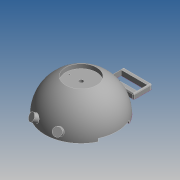
# Autodesk Inventor part: body_face
Saved by Autodesk Inventor 2017 (Build 210142000, 142)
## iProperties
Created: 2018-10-05
Part Number: body_face
Material: Générique
Document SubType Name: Modeling
Designer: Gilles Mottiez
Density: 1 g/cm^3
Appearance: Par défaut
Author: Gilles Mottiez
Autodesk Inventor part; units mm, degrees
ref_plane "YZ Plane" through (0, 0, 0) normal (1, 0, 0) x (0, 1, 0)
ref_plane "XZ Plane" through (0, 0, 0) normal (0, 1, 0) x (-1, 0, 0)
ref_plane "XY Plane" through (0, 0, 0) normal (0, 0, 1) x (1, 0, 0)
sketch "Sketch1" plane through (0, 0, 0) normal (0, 0, 1) x (1, 0, 0)
  circle A0 centre (0, 0) radius 70 construction
  line L0 (-70, 0) -> (70, 0) construction
  arc A1 (70, 0) -> (-70, 0) centre (0, 0) ccw
  line L1 (-70, 0) -> (70, 0)
  dimension "d0" = 140
  constraints: 4 end point, 4 point on circle, 2 centre point, 2 coincident, 1 collinear, 1 concentric, 1 horizontal, 1 midpoint
  measures "d0" diameter of A0
revolve "Révolution1" add sketch "Sketch1" angle 180 about axis through (-70, 0, 0) along (1, 0, 0)
sketch "Esquisse2" plane through (0, 0, 0) normal (1, 0, 0) x (0, 1, 0)
  line L0 (-70, 0) -> (70, 0) construction
  circle A0 centre (0, 0) radius 67 construction
  arc A1 (67, 0) -> (-67, 0) centre (0, 0) ccw
  line L1 (67, 0) -> (-67, 0)
  dimension "d2" = 134
  constraints: 4 point on circle, 2 centre point, 2 concentric, 2 end point, 2 point on line, 1 coincident, 1 collinear
  measures "d2" diameter of A0
revolve "Révolution2" cut sketch "Esquisse2" angle 360 about axis through (0, 67, 0) along (0, -1, 0)
sketch "Esquisse3" plane through (0, 0, 0) normal (1, 0, 0) x (0, 1, 0)
  line L0 (67, 0) -> (-67, 0) construction
  line L1 (-70, 0) -> (70, 0) construction
  arc A0 (70, 0) -> (-70, 0) centre (0, 0) ccw construction
  line L2 (30, 0) -> (-30, 0)
  line L3 (-30, 0) -> (-30, 5.5)
  line L4 (-30, 5.5) -> (30, 5.5)
  line L5 (30, 5.5) -> (30, 0)
  point P0 (0, 0)
  point P1 (0, 0)
  point P2 (0, 5.5)
  dimension "d4" = 60
  dimension "d5" = 5.5
  constraints: 8 end point, 2 midpoint, 2 parallel, 1 horizontal, 1 perpendicular, 1 point on line, 1 vertical alignment
  measures "d4" distance of L3.end L4.end
  measures "d5" distance of L4.end L2.start
extrude "Extrusion1" cut sketch "Esquisse3" along normal through all both and the other way through all
sketch "Esquisse4" plane through (0, 0, 0) normal (0, 0, -1) x (-1, 0, 0)
  line L0 (-63.2456, 30) -> (-59.9083, 30) construction
  arc A0 (59.9083, 30) -> (-59.9083, 30) centre (0, 0) ccw construction
  line L1 (59.9083, 30) -> (63.2456, 30) construction
  arc A1 (63.2456, 30) -> (-63.2456, 30) centre (0, 0) ccw construction
  arc A2 (-59.9083, -30) -> (59.9083, -30) centre (0, 0) ccw construction
  line L2 (-59.9083, -30) -> (-63.2456, -30) construction
  arc A3 (-63.2456, -30) -> (63.2456, -30) centre (0, 0) ccw construction
  line L3 (63.2456, -30) -> (59.9083, -30) construction
  arc A4 (-59.9083, -30) -> (59.9083, -30) centre (0, 0) ccw construction
  arc A5 (-59.6553, 30) -> (-59.6553, -30) centre (0, 0) ccw construction
  line L4 (-63.006, 30) -> (-59.6553, 30) construction
  arc A6 (-63.006, 30) -> (-63.006, -30) centre (0, 0) ccw construction
  line L5 (-63.006, -30) -> (-59.6553, -30) construction
  arc A7 (59.6553, -30) -> (59.6553, 30) centre (0, 0) ccw construction
  line L6 (59.6553, -30) -> (63.006, -30) construction
  arc A8 (63.006, -30) -> (63.006, 30) centre (0, 0) ccw construction
  line L7 (59.6553, 30) -> (63.006, 30) construction
  line L8 (0, 0) -> (-49.4975, 49.4975) construction
  line L9 (0, 0) -> (-69.7836, 0) construction
  circle A9 centre (0, 0) radius 63 construction
  circle A10 centre (-44.5477, 44.5477) radius 4 construction
  line L10 (-41.6309, 47.2849) -> (-44.5602, 50.0339)
  line L11 (-47.2849, 41.6309) -> (-50.2031, 44.3694)
  arc A11 (-44.5602, 50.0339) -> (-50.2031, 44.3694) centre (0, 0) ccw
  arc A12 (-47.2849, 41.6309) -> (-41.6309, 47.2849) centre (-44.5477, 44.5477) ccw
  dimension "d8" = 45
  dimension "d9" = 126
  dimension "d10" = 8
  constraints: 13 point on circle, 8 end point, 4 centre point, 2 concentric, 2 tangent, 1 coincident, 1 parallel, 1 point on line
  measures "d8" angle of L8 L9
  measures "d9" diameter of A9
  measures "d10" diameter of A10
extrude "Extrusion2" add sketch "Esquisse4" against normal up to surface
pattern_circular "Réseau circulaire1" count 4 over 360 about axis through (0, 0, 0) along (0, 0, 1) of "Extrusion2"
sketch "Esquisse6" plane through (0, 0, 0) normal (0, 0, -1) x (-1, 0, 0)
  line L0 (-63.2456, 30) -> (-59.9083, 30) construction
  arc A0 (-50.2031, 44.3694) -> (-59.9083, 30) centre (0, 0) ccw construction
  line L1 (-50.2031, 44.3694) -> (-47.2849, 41.6309) construction
  arc A1 (-47.2849, 41.6309) -> (-41.6309, 47.2849) centre (-44.5477, 44.5477) ccw construction
  line L2 (-41.6309, 47.2849) -> (-44.5602, 50.0339) construction
  arc A2 (44.3694, 50.2031) -> (-44.5602, 50.0339) centre (0, 0) ccw construction
  line L3 (44.3694, 50.2031) -> (41.6309, 47.2849) construction
  arc A3 (41.6309, 47.2849) -> (47.2849, 41.6309) centre (44.5477, 44.5477) ccw construction
  line L4 (47.2849, 41.6309) -> (50.0339, 44.5602) construction
  arc A4 (59.9083, 30) -> (50.0339, 44.5602) centre (0, 0) ccw construction
  line L5 (59.9083, 30) -> (63.2456, 30) construction
  arc A5 (63.2456, 30) -> (-63.2456, 30) centre (0, 0) ccw construction
  circle A6 centre (-44.5477, 44.5477) radius 2.5
  dimension "d19" = 5
  constraints: 1 centre point, 1 coincident
  measures "d19" diameter of A6
extrude "Extrusion4" cut sketch "Esquisse6" against normal blind 4
pattern_circular "Réseau circulaire2" count 4 over 360 about axis through (0, 0, 0) along (0, 0, 1) of "Extrusion4"
sketch "Esquisse7" plane through (0, 0, 0) normal (0, 0, 1) x (1, 0, 0)
  arc A0 (-63.2456, -30) -> (63.2456, -30) centre (0, 0) ccw construction
  line L0 (50.0339, -44.5602) -> (47.2849, -41.6309) construction
  line L1 (41.6309, -47.2849) -> (44.3694, -50.2031) construction
  arc A1 (-44.5602, -50.0339) -> (44.3694, -50.2031) centre (0, 0) ccw construction
  line L2 (-44.5602, -50.0339) -> (-41.6309, -47.2849) construction
  line L3 (-47.2849, -41.6309) -> (-50.2031, -44.3694) construction
  arc A2 (-59.9083, -30) -> (-50.2031, -44.3694) centre (0, 0) ccw construction
  line L4 (-59.9083, -30) -> (-59.6553, -30) construction
  arc A3 (-59.6553, 30) -> (-59.6553, -30) centre (0, 0) ccw construction
  line L5 (-59.6553, 30) -> (-59.9083, 30) construction
  arc A4 (-50.0339, 44.5602) -> (-59.9083, 30) centre (0, 0) ccw construction
  line L6 (-50.0339, 44.5602) -> (-47.2849, 41.6309) construction
  line L7 (-41.6309, 47.2849) -> (-44.3694, 50.2031) construction
  arc A5 (44.5602, 50.0339) -> (-44.3694, 50.2031) centre (0, 0) ccw construction
  line L8 (44.5602, 50.0339) -> (41.6309, 47.2849) construction
  line L9 (47.2849, 41.6309) -> (50.2031, 44.3694) construction
  arc A6 (59.9083, 30) -> (50.2031, 44.3694) centre (0, 0) ccw construction
  line L10 (59.9083, 30) -> (59.6553, 30) construction
  arc A7 (59.6553, -30) -> (59.6553, 30) centre (0, 0) ccw construction
  line L11 (59.6553, -30) -> (59.9083, -30) construction
  arc A8 (50.0339, -44.5602) -> (59.9083, -30) centre (0, 0) ccw construction
  line L12 (50, -70) -> (-50, -70) construction
  point P0 (0, -70)
  point P1 (0, -70)
  dimension "d25" = 100
  constraints: 2 end point, 1 coincident, 1 horizontal, 1 midpoint, 1 point on circle, 1 vertical alignment, 4 other
  measures "d25" distance of L12.start L12.end
ref_plane "Plan de construction1" through (50, -70, 0) normal (0, -0.8660254, 0.5) x (-1, 0, 0)
ref_plane "Plan de construction2" through (50, -78.6603, 5) normal (0, -0.8660254, 0.5) x (-1, 0, 0)
sketch "Esquisse9" plane through (50, -78.6603, 5) normal (0, -0.8660254, 0.5) x (-1, 0, 0)
  line L0 (0, 0) -> (100, 0) construction
  ellipse E0 centre (50, -50) end of major axis (113.2456, -50) minor radius 54.7723 (-13.2456, -50) -> (-13.006, -54.7631) ccw construction
  ellipse E1 centre (50, -35) end of major axis (120, -35) minor radius 35 (-13.2456, -50) -> (113.2456, -50) ccw construction
  ellipse E2 centre (50, -50) end of major axis (113.2456, -50) minor radius 54.7723 (113.006, -54.7631) -> (113.2456, -50) ccw construction
  ellipse E3 centre (50, -39.7631) end of major axis (119.7836, -39.7631) minor radius 34.8918 (113.006, -54.7631) -> (113.006, -24.7631) ccw construction
  ellipse E4 centre (50, -20) end of major axis (113.2456, -20) minor radius 54.7723 (113.006, -24.7631) -> (113.2456, -20) ccw construction
  ellipse E5 centre (50, -35) end of major axis (120, -35) minor radius 35 (113.2456, -20) -> (-13.2456, -20) ccw construction
  ellipse E6 centre (50, -20) end of major axis (113.2456, -20) minor radius 54.7723 (-13.2456, -20) -> (-13.006, -24.7631) ccw construction
  ellipse E7 centre (50, -39.7631) end of major axis (119.7836, -39.7631) minor radius 34.8918 (-13.006, -24.7631) -> (-13.006, -54.7631) ccw construction
  line L1 (75, 0) -> (75, -50) construction
  line L2 (25, 0) -> (25, -50) construction
  point P0 (50, -35)
  point P1 (50, 0)
  dimension "d32" = 50
  dimension "d34" = 25
  dimension "d40" = 50
  dimension "d41" = 25
  constraints: 4 end point, 2 point on line, 2 vertical, 8 other
  measures "d32" distance of L1.start L1.end
  measures "d34" distance from line of point (50, 0) L1
  measures "d40" distance of L2.start L2.end
  measures "d41" distance from line of L2 point (50, -20)
ref_plane "Plan de construction3" through (-25, -78.6603, 5) normal (-0.3420201, -0.8137977, 0.4698463) x (0, 0.5, 0.8660254)
sketch "Esquisse10" plane through (-25, -78.6603, 5) normal (-0.3420201, -0.8137977, 0.4698463) x (0, 0.5, 0.8660254)
  ellipse E0 centre (50, 9.5477) end of major axis (17.7652, 63.962) minor radius 51.4691 (50, -49.8837) -> (54.7631, -50.5991) ccw construction
  ellipse E1 centre (35, 0.6618) end of major axis (48.5607, 69.3357) minor radius 32.8892 (50, -49.8837) -> (50, 68.9791) ccw construction
  ellipse E2 centre (50, 9.5477) end of major axis (17.7652, 63.962) minor radius 51.4691 (54.7631, 67.8134) -> (50, 68.9791) ccw construction
  ellipse E3 centre (39.7631, -0.2788) end of major axis (53.2819, 68.1828) minor radius 32.7876 (54.7631, 67.8134) -> (24.7631, 50.0415) ccw construction
  ellipse E4 centre (20, -8.2242) end of major axis (-12.2348, 46.1901) minor radius 51.4691 (24.7631, 50.0415) -> (20, 51.2072) ccw construction
  ellipse E5 centre (35, 0.6618) end of major axis (48.5607, 69.3357) minor radius 32.8892 (20, 51.2072) -> (20, -67.6556) ccw construction
  ellipse E6 centre (20, -8.2242) end of major axis (-12.2348, 46.1901) minor radius 51.4691 (20, -67.6556) -> (24.7631, -68.371) ccw construction
  ellipse E7 centre (39.7631, -0.2788) end of major axis (53.2819, 68.1828) minor radius 32.7876 (24.7631, -68.371) -> (54.7631, -50.5991) ccw construction
  line L0 (0, 0) -> (50, 0) construction
  line L1 (0, -70.4769) -> (0, 23.4923) construction
  circle A0 centre (15, 0) radius 7.5
  point P0 (35, 0.6618)
  dimension "d36" = 15
  dimension "d37" = 15
  constraints: 1 centre point, 1 point on line, 8 other
  measures "d36" diameter of A0
  measures "d37" distance from line of L1 A0.centre
extrude "Extrusion5" add sketch "Esquisse10" against normal up to surface
ref_plane "Plan de construction4" through (25, -78.6603, 5) normal (0.3420201, -0.8137977, 0.4698463) x (0, 0.5, 0.8660254)
sketch "Esquisse11" plane through (25, -78.6603, 5) normal (0.3420201, -0.8137977, 0.4698463) x (0, 0.5, 0.8660254)
  line L0 (0, 0) -> (50, 0) construction
  line L1 (0, -23.4923) -> (0, 70.4769) construction
  circle A0 centre (15, 0) radius 7.5
  point P0 (35, -0.6618)
  dimension "d43" = 15
  dimension "d44" = 15
  constraints: 1 centre point, 1 point on line
  measures "d43" diameter of A0
  measures "d44" distance from line of L1 A0.centre
extrude "Extrusion6" add sketch "Esquisse11" against normal up to surface
sketch "Esquisse12" plane through (0, 0, 0) normal (1, 0, 0) x (0, 1, 0)
  arc A0 (67, 0) -> (-67, 0) centre (0, 0) ccw construction
  arc A1 (70, 0) -> (-70, 0) centre (0, 0) ccw construction
  line L0 (0, -14.3596) -> (0, 86.1577) construction
  ellipse E0 centre (4.1003, 0) end of major axis (4.1003, -66.7315) minor radius 48.6605 (-41.6309, 22.8035) -> (-44.5602, 0) ccw construction
  ellipse E1 centre (-1.3686, 0) end of major axis (-1.3686, 66.9701) minor radius 48.8345 (-47.2849, 22.8035) -> (-50.2031, 0) ccw construction
  line L1 (-50.0339, 0) -> (-50.2031, 0) construction
  ellipse E2 centre (-4.3693, 0) end of major axis (-4.3693, 66.7315) minor radius 45.6646 (-47.2849, 22.8035) -> (-50.0339, 0) ccw construction
  ellipse E3 centre (1.4584, 0) end of major axis (1.4584, -66.9701) minor radius 45.8278 (-41.6309, 22.8035) -> (-44.3694, 0) ccw construction
  line L2 (-30, 0) -> (-44.3694, 0) construction
  line L3 (-30, 0) -> (-30, 5.5) construction
  line L4 (-30, 5.5) -> (30, 5.5) construction
  line L5 (30, 5.5) -> (30, 0) construction
  line L6 (44.5602, 0) -> (30, 0) construction
  ellipse E4 centre (-4.1003, 0) end of major axis (-4.1003, 66.7315) minor radius 48.6605 (44.5602, 0) -> (41.6309, 22.8035) ccw construction
  ellipse E5 centre (1.3686, 0) end of major axis (1.3686, -66.9701) minor radius 48.8345 (50.2031, 0) -> (47.2849, 22.8035) ccw construction
  line L7 (50.0339, 0) -> (50.2031, 0) construction
  ellipse E6 centre (4.3693, 0) end of major axis (4.3693, -66.7315) minor radius 45.6646 (50.0339, 0) -> (47.2849, 22.8035) ccw construction
  ellipse E7 centre (-1.4584, 0) end of major axis (-1.4584, 66.9701) minor radius 45.8278 (44.3694, 0) -> (41.6309, 22.8035) ccw construction
  line L8 (30, 0) -> (44.3694, 0) construction
  line L9 (30, 0) -> (30, 5.5) construction
  line L10 (30, 5.5) -> (-30, 5.5) construction
  line L11 (-30, 5.5) -> (-30, 0) construction
  line L12 (-44.5602, 0) -> (-30, 0) construction
  line L13 (0, 47) -> (47.7493, 47)
  arc A2 (47.7493, 47) -> (0, 67) centre (0, 0) ccw
  line L14 (0, 67) -> (0, 47)
  point P0 (0, 0)
  point P1 (4, 66.8805)
  point P2 (-4, 66.8805)
  dimension "d48" = 20
  constraints: 4 end point, 4 horizontal alignment, 4 point on circle, 2 point on line, 1 centre point, 1 collinear, 1 concentric, 1 horizontal, 8 other
  measures "d48" distance from line of L14.start L13
revolve "Révolution3" add sketch "Esquisse12" angle 360 about axis through (0, 0, 67) along (0, 0, -1)
sketch "Esquisse13" plane through (0, 0, 0) normal (1, 0, 0) x (0, 1, 0)
  line L0 (30, 5.5) -> (30, 0) construction
  line L1 (30, 0) -> (30, 0) construction
  line L2 (30, 0) -> (30, 5.5) construction
  line L3 (30, 5.5) -> (-30, 5.5) construction
  line L4 (-30, 5.5) -> (-30, 0) construction
  line L5 (-30, 0) -> (-30, 0) construction
  line L6 (-30, 0) -> (-30, 5.5) construction
  line L7 (-30, 5.5) -> (30, 5.5) construction
  line L8 (47.7493, 47) -> (-47.7493, 47) construction
  line L9 (0, -15) -> (0, 90) construction
  arc A0 (70, 0) -> (-70, 0) centre (0, 0) ccw construction
  line L10 (0, 55) -> (30, 55) construction
  line L11 (30, 55) -> (30, 75) construction
  line L12 (30, 75) -> (0, 75) construction
  line L13 (0, 75) -> (0, 55) construction
  line L14 (0, 55) -> (30, 55)
  line L15 (30, 55) -> (30, 63.2456)
  arc A1 (30, 63.2456) -> (0, 70) centre (0, 0) ccw
  line L16 (0, 55) -> (0, 70)
  point P0 (0, 0)
  dimension "d50" = 8
  dimension "d51" = 30
  dimension "d52" = 20
  constraints: 14 end point, 4 point on circle, 3 point on line, 2 collinear, 2 parallel, 1 centre point, 1 concentric, 1 horizontal, 1 perpendicular, 2 other
  measures "d50" distance between parallel lines of L10 L8
  measures "d51" distance between parallel lines of L13 L11
  measures "d52" distance of L10.end L11.end
revolve "Révolution4" cut sketch "Esquisse13" angle 360 about axis through (0, 0, 55) along (0, 0, 1)
sketch "Esquisse15" plane through (0, 0, 55) normal (0, 0, 1) x (1, 0, 0)
  point P0 (0, 0)
  point P1 (-23, 0)
  dimension "d57" = 23
  constraints: 1 horizontal alignment
  measures "d57" distance of point (-23, 0) point (0, 0)
hole "Perçage1" at (-23, 0, 55) direction (0, 0, -1) diameter 3 depth 8 tip angle 118
sketch "Esquisse16" plane through (0, 0, 0) normal (1, 0, 0) x (0, 1, 0)
  line L0 (-30, 63.2456) -> (30, 63.2456) construction
  line L1 (30, 5.5) -> (30, 0) construction
  line L2 (30, 0) -> (30, 0) construction
  line L3 (30, 0) -> (30, 5.5) construction
  line L4 (30, 5.5) -> (-30, 5.5) construction
  line L5 (-30, 5.5) -> (-30, 0) construction
  line L6 (-30, 0) -> (-30, 0) construction
  line L7 (-30, 0) -> (-30, 5.5) construction
  line L8 (-30, 5.5) -> (30, 5.5) construction
  line L9 (47.7493, 47) -> (-47.7493, 47) construction
  line L10 (4, 47) -> (-4, 47) construction
  line L11 (-4, 55) -> (4, 55) construction
  line L12 (0, -13.1244) -> (0, 78.7461) construction
  line L13 (0, 41) -> (6, 41) construction
  line L14 (6, 41) -> (6, 47) construction
  line L15 (6, 47) -> (0, 47) construction
  line L16 (0, 47) -> (0, 41) construction
  arc A0 (11, 47) -> (6, 42) centre (11, 42) ccw construction
  line L17 (0, 47) -> (11, 47)
  line L18 (6, 41) -> (0, 41)
  line L19 (6, 41) -> (6, 42)
  arc A1 (11, 47) -> (6, 42) centre (11, 42) ccw
  line L20 (0, 41) -> (0, 47)
  point P0 (0, 0)
  dimension "d65" = 12
  dimension "d67" = 5
  dimension "d68" = 6
  constraints: 16 end point, 4 collinear, 4 point on circle, 4 point on line, 3 tangent, 2 centre point, 2 parallel, 1 concentric, 1 horizontal, 1 perpendicular, 2 other
  measures "d65" diameter of L14 L20
  measures "d67" radius of A0
  measures "d68" distance between parallel lines of L17 L13
revolve "Révolution5" add sketch "Esquisse16" angle 360 about axis through (0, 0, 41) along (0, 0, 1)
sketch "Esquisse17" plane through (0, 0, 41) normal (0, 0, -1) x (-1, 0, 0)
  circle A0 centre (0, 0) radius 4
  point P0 (0, 0)
  dimension "d70" = 8
  constraints: 1 centre point, 1 coincident
  measures "d70" diameter of A0
extrude "Extrusion8" cut sketch "Esquisse17" against normal through all
sketch "Esquisse19" plane through (0, 0, 0) normal (0, 0, -1) x (-1, 0, 0)
  circle A0 centre (44.5477, 44.5477) radius 2.5 construction
  circle A1 centre (-44.5477, 44.5477) radius 2.5 construction
  line L0 (-63.2456, 30) -> (-59.9083, 30) construction
  arc A2 (-50.2031, 44.3694) -> (-59.9083, 30) centre (0, 0) ccw construction
  line L1 (-50.2031, 44.3694) -> (-47.2849, 41.6309) construction
  arc A3 (-47.2849, 41.6309) -> (-41.6309, 47.2849) centre (-44.5477, 44.5477) ccw construction
  line L2 (-41.6309, 47.2849) -> (-44.5602, 50.0339) construction
  arc A4 (44.3694, 50.2031) -> (-44.5602, 50.0339) centre (0, 0) ccw construction
  line L3 (44.3694, 50.2031) -> (41.6309, 47.2849) construction
  arc A5 (41.6309, 47.2849) -> (47.2849, 41.6309) centre (44.5477, 44.5477) ccw construction
  line L4 (47.2849, 41.6309) -> (50.0339, 44.5602) construction
  arc A6 (59.9083, 30) -> (50.0339, 44.5602) centre (0, 0) ccw construction
  line L5 (59.9083, 30) -> (63.2456, 30) construction
  arc A7 (63.2456, 30) -> (-63.2456, 30) centre (0, 0) ccw construction
  line L6 (0, 0) -> (0, 70) construction
  line L7 (-27.5, 110) -> (27.5, 110) construction
  line L8 (27.5, 110) -> (27.5, 75) construction
  line L9 (27.5, 75) -> (-27.5, 75) construction
  line L10 (-27.5, 75) -> (-27.5, 110) construction
  line L11 (-10, 75) -> (10, 75) construction
  line L12 (10, 75) -> (10, 69.282) construction
  line L13 (10, 69.282) -> (-10, 69.282) construction
  line L14 (-10, 69.282) -> (-10, 75) construction
  line L15 (-10, 69.282) -> (-10, 75)
  line L16 (-10, 75) -> (-27.5, 75)
  line L17 (-27.5, 75) -> (-27.5, 110)
  line L18 (-27.5, 110) -> (27.5, 110)
  line L19 (27.5, 110) -> (27.5, 75)
  line L20 (27.5, 75) -> (10, 75)
  line L21 (10, 75) -> (10, 69.282)
  line L22 (10, 69.282) -> (-10, 69.282)
  dimension "d79" = 55
  dimension "d80" = 35
  dimension "d81" = 75
  dimension "d82" = 20
  constraints: 34 end point, 7 collinear, 4 parallel, 3 horizontal, 2 perpendicular, 2 point on circle, 1 point on line, 2 other
  measures "d79" distance of L8.end L9.end
  measures "d80" distance of L7.end L8.end
  measures "d81" distance from line of point (0, 0) L9
  measures "d82" distance of L12.end L13.end
extrude "Extrusion10" add sketch "Esquisse19" against normal blind 10
thicken "Epaississement2" operation add thickness 1 both sides no extend neighbours yes toward (0, -1, 0) faces at (8.0177, 69.282, 8.0177)
thicken "Epaississement3" operation add thickness 1 both sides no extend neighbours yes toward (0, -1, 0) faces at (-8.0177, 69.282, 8.0177)
fillet "Congé1" radius 2 14 edges at (10, 71.7783, 10) (10, 69.1004, 5.0131) (-10, 71.7783, 10) (0, 69.282, 10) (-10, 69.1004, 5.0131) (-18.75, 75, 10) (-27.5, 92.5, 10) (0, 110, 10) (27.5, 92.5, 10) (18.75, 75, 10) (27.5, 110, 5) (-27.5, 110, 5) (27.5, 75, 5) (-27.5, 75, 5)
sketch "Esquisse20" plane through (25.5, 110, 0) normal (0, 0, -1) x (-1, 0, 0)
  arc A0 (0, 0) -> (-2, -2) centre (0, -2) ccw construction
  line L0 (-2, -2) -> (-2, -33) construction
  arc A1 (-2, -33) -> (0, -35) centre (0, -33) ccw construction
  line L1 (0, -35) -> (15.5, -35) construction
  line L2 (15.5, -35) -> (15.5, -39.007) construction
  arc A2 (13.8333, -40.9791) -> (15.5, -39.007) centre (13.5, -39.007) ccw construction
  arc A3 (13.8333, -40.9791) -> (-37.7456, -80) centre (25.5, -110) ccw construction
  line L3 (-37.7456, -80) -> (-34.4083, -80) construction
  arc A4 (-24.7031, -65.6306) -> (-34.4083, -80) centre (25.5, -110) ccw construction
  line L4 (-24.7031, -65.6306) -> (-21.7849, -68.3691) construction
  arc A5 (-21.7849, -68.3691) -> (-16.1309, -62.7151) centre (-19.0477, -65.4523) ccw construction
  line L5 (-16.1309, -62.7151) -> (-19.0602, -59.9661) construction
  arc A6 (69.8694, -59.7969) -> (-19.0602, -59.9661) centre (25.5, -110) ccw construction
  line L6 (69.8694, -59.7969) -> (67.1309, -62.7151) construction
  arc A7 (67.1309, -62.7151) -> (72.7849, -68.3691) centre (70.0477, -65.4523) ccw construction
  line L7 (72.7849, -68.3691) -> (75.5339, -65.4398) construction
  arc A8 (85.4083, -80) -> (75.5339, -65.4398) centre (25.5, -110) ccw construction
  line L8 (85.4083, -80) -> (88.7456, -80) construction
  arc A9 (88.7456, -80) -> (37.1667, -40.9791) centre (25.5, -110) ccw construction
  arc A10 (35.5, -39.007) -> (37.1667, -40.9791) centre (37.5, -39.007) ccw construction
  line L9 (35.5, -39.007) -> (35.5, -35) construction
  line L10 (35.5, -35) -> (51, -35) construction
  arc A11 (51, -35) -> (53, -33) centre (51, -33) ccw construction
  line L11 (53, -33) -> (53, -2) construction
  arc A12 (53, -2) -> (51, 0) centre (51, -2) ccw construction
  line L12 (51, 0) -> (0, 0) construction
  circle A13 centre (-19.0477, -65.4523) radius 2.5 construction
  circle A14 centre (70.0477, -65.4523) radius 2.5 construction
  line L13 (0, -7) -> (51, -7)
  line L14 (51, -7) -> (51, -27)
  line L15 (51, -27) -> (0, -27)
  line L16 (0, -27) -> (0, -7)
  line L17 (25.5, 0) -> (25.5, -43) construction
  dimension "d90" = 51
  dimension "d91" = 20
  dimension "d92" = 7
  constraints: 10 end point, 2 parallel, 1 horizontal, 1 midpoint, 1 perpendicular, 1 point on circle, 1 vertical, 1 other
  measures "d90" distance of L14.end L15.end
  measures "d91" distance of L13.end L14.end
  measures "d92" distance between parallel lines of L12 L13
extrude "Extrusion11" cut sketch "Esquisse20" against normal through all
sketch "Esquisse21" plane through (25.5, 110, 0) normal (0, 0, -1) x (-1, 0, 0)
  line L0 (0, -27) -> (0, -7) construction
  line L1 (0, -7) -> (51, -7) construction
  line L2 (51, -7) -> (51, -27) construction
  line L3 (51, -27) -> (0, -27) construction
  arc A0 (0, 0) -> (-2, -2) centre (0, -2) ccw construction
  line L4 (-2, -2) -> (-2, -33) construction
  arc A1 (-2, -33) -> (0, -35) centre (0, -33) ccw construction
  line L5 (0, -35) -> (15.5, -35) construction
  line L6 (15.5, -35) -> (15.5, -39.007) construction
  arc A2 (13.8333, -40.9791) -> (15.5, -39.007) centre (13.5, -39.007) ccw construction
  arc A3 (13.8333, -40.9791) -> (-37.7456, -80) centre (25.5, -110) ccw construction
  line L7 (-37.7456, -80) -> (-34.4083, -80) construction
  arc A4 (-24.7031, -65.6306) -> (-34.4083, -80) centre (25.5, -110) ccw construction
  line L8 (-24.7031, -65.6306) -> (-21.7849, -68.3691) construction
  arc A5 (-21.7849, -68.3691) -> (-16.1309, -62.7151) centre (-19.0477, -65.4523) ccw construction
  line L9 (-16.1309, -62.7151) -> (-19.0602, -59.9661) construction
  arc A6 (69.8694, -59.7969) -> (-19.0602, -59.9661) centre (25.5, -110) ccw construction
  line L10 (69.8694, -59.7969) -> (67.1309, -62.7151) construction
  arc A7 (67.1309, -62.7151) -> (72.7849, -68.3691) centre (70.0477, -65.4523) ccw construction
  line L11 (72.7849, -68.3691) -> (75.5339, -65.4398) construction
  arc A8 (85.4083, -80) -> (75.5339, -65.4398) centre (25.5, -110) ccw construction
  line L12 (85.4083, -80) -> (88.7456, -80) construction
  arc A9 (88.7456, -80) -> (37.1667, -40.9791) centre (25.5, -110) ccw construction
  arc A10 (35.5, -39.007) -> (37.1667, -40.9791) centre (37.5, -39.007) ccw construction
  line L13 (35.5, -39.007) -> (35.5, -35) construction
  line L14 (35.5, -35) -> (51, -35) construction
  arc A11 (51, -35) -> (53, -33) centre (51, -33) ccw construction
  line L15 (53, -33) -> (53, -2) construction
  arc A12 (53, -2) -> (51, 0) centre (51, -2) ccw construction
  line L16 (51, 0) -> (0, 0) construction
  circle A13 centre (-19.0477, -65.4523) radius 2.5 construction
  circle A14 centre (70.0477, -65.4523) radius 2.5 construction
